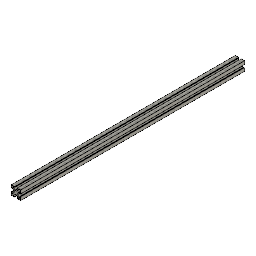
Frame Assembly v7 (Autodesk Fusion 360 archive; units mm, degrees)
design "TS10-10"
Autodesk Fusion 360 part; units mm, degrees
sketch "Sketch1" plane through (0, 0, 0) normal (0, 1, 0) x (1, 0, 0)
  line L0 (0, 0) -> (0, 4.826)
  line L1 (0, 4.826) -> (2, 4.826)
  line L2 (2, 4.826) -> (7.874, 10.7)
  line L3 (7.874, 10.7) -> (3.302, 10.7)
  line L4 (3.302, 10.7) -> (3.302, 12.7)
  line L5 (3.302, 12.7) -> (12.7, 12.7)
  line L6 (12.7, 12.7) -> (12.7, 3.302)
  line L7 (12.7, 3.302) -> (10.7, 3.302)
  line L8 (10.7, 3.302) -> (10.7, 7.874)
  line L9 (10.7, 7.874) -> (4.826, 2)
  line L10 (4.826, 2) -> (4.826, 0)
  line L11 (4.826, 0) -> (0, 0)
  line L12 (0, 4.826) -> (-2, 4.826)
  line L13 (-4.826, 2) -> (-4.826, 0)
  line L14 (-7.874, 10.7) -> (-3.302, 10.7)
  line L15 (-10.7, 3.302) -> (-10.7, 7.874)
  line L16 (-4.826, 0) -> (0, 0)
  line L17 (-12.7, 3.302) -> (-10.7, 3.302)
  line L18 (-3.302, 10.7) -> (-3.302, 12.7)
  line L19 (-2, 4.826) -> (-7.874, 10.7)
  line L20 (-12.7, 12.7) -> (-12.7, 3.302)
  line L21 (-3.302, 12.7) -> (-12.7, 12.7)
  line L22 (-10.7, 7.874) -> (-4.826, 2)
  line L23 (0, -4.826) -> (2, -4.826)
  line L24 (12.7, -3.302) -> (10.7, -3.302)
  line L25 (7.874, -10.7) -> (3.302, -10.7)
  line L26 (3.302, -10.7) -> (3.302, -12.7)
  line L27 (3.302, -12.7) -> (12.7, -12.7)
  line L28 (-12.7, -3.302) -> (-10.7, -3.302)
  line L29 (10.7, -7.874) -> (4.826, -2)
  line L30 (-10.7, -7.874) -> (-4.826, -2)
  line L31 (-10.7, -3.302) -> (-10.7, -7.874)
  line L32 (-12.7, -12.7) -> (-12.7, -3.302)
  line L33 (12.7, -12.7) -> (12.7, -3.302)
  line L34 (4.826, -2) -> (4.826, 0)
  line L35 (2, -4.826) -> (7.874, -10.7)
  line L36 (10.7, -3.302) -> (10.7, -7.874)
  line L37 (0, -4.826) -> (-2, -4.826)
  line L38 (-7.874, -10.7) -> (-3.302, -10.7)
  line L39 (-4.826, -2) -> (-4.826, 0)
  line L40 (-3.302, -10.7) -> (-3.302, -12.7)
  line L41 (0, 0) -> (0, -4.826)
  line L42 (-2, -4.826) -> (-7.874, -10.7)
  line L43 (-3.302, -12.7) -> (-12.7, -12.7)
  dimension "d1" = 12.7
  dimension "d2" = 12.7
  dimension "d3" = 3.302
  dimension "d4" = 3.302
  dimension "d5" = 7.874
  dimension "d6" = 7.874
  dimension "d8" = 7.874
  dimension "d9" = 2
  dimension "d10" = 2
  constraint coincident L0.start L11.end
  constraint vertical L0
  constraint perpendicular L0 L1
  constraint perpendicular L3 L4
  constraint perpendicular L4 L5
  constraint perpendicular L5 L6
  constraint perpendicular L4 L7
  constraint perpendicular L0 L11
  constraint vertical L10
  constraint coincident L3.end L4.start
  constraint coincident L7.end L8.start
  constraint vertical L8
  constraint equal L3 L8
  constraint parallel L2 L9
  constraint equal L1 L10
  constraint symmetric L11.end L0 L16.end
  constraint symmetric L1.start L0 L12.start
  constraint symmetric L0 L1.end L12.end
  constraint symmetric L0 L2.end L14.start
  constraint symmetric L0 L3.end L14.end
  constraint symmetric L0 L4.end L18.end
  constraint symmetric L0 L5.end L20.start
  constraint symmetric L0 L6.end L17.start
  constraint symmetric L0 L7.end L15.start
  constraint symmetric L0 L8.end L15.end
  constraint symmetric L0 L9.end L13.start
  constraint symmetric L0 L10.end L13.end
  constraint symmetric L0.start L11 L16.end
  constraint symmetric L0.end L11 L23.start
  constraint symmetric L1.end L11 L23.end
  constraint symmetric L2.end L11 L25.start
  constraint symmetric L3.end L11 L25.end
  constraint symmetric L4.end L11 L26.end
  constraint symmetric L5.end L11 L27.end
  constraint symmetric L6.end L11 L24.start
  constraint symmetric L7.end L11 L24.end
  constraint symmetric L8.end L11 L29.start
  constraint symmetric L9.end L11 L29.end
  constraint symmetric L10.end L11 L34.end
  constraint symmetric L11 L0.start L16.end
  constraint symmetric L11 L0.end L23.start
  constraint symmetric L11 L12.end L37.end
  constraint symmetric L11 L15.start L28.end
  constraint symmetric L11 L15.end L30.start
  constraint symmetric L11 L17.start L28.start
  constraint symmetric L11 L20.start L32.start
  constraint symmetric L11 L13.end L16.start
  constraint symmetric L11 L13.start L30.end
  constraint symmetric L11 L18.end L40.end
  constraint symmetric L11 L14.start L38.start
  constraint symmetric L11 L14.end L38.end
  measures "d1" horizontal distance of L0.start L5.end
  measures "d2" vertical distance of L0.start L5.end
  measures "d3" horizontal distance of L0.start L4.end
  measures "d4" vertical distance of L0.start L6.end
  measures "d5" distance of L1 L5
  measures "d6" distance of L6 L10
  measures "d8" horizontal distance of L0.start L2.end
  measures "d9" distance of L3.end L4.end
  measures "d10" distance of L6.end L7.end
extrude "Extrude1" add sketch "Sketch1" along normal blind 609.33
equation "d2 = d1"
equation "d3 = 0.26 in / 2"
equation "d4 = d3"
equation "d8 = 0.62 in / 2"

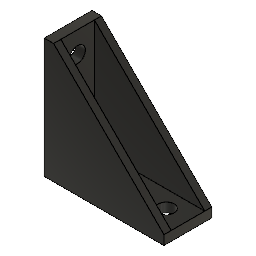
design "Small Bracket"
Autodesk Fusion 360 part; units mm, degrees
sketch "Sketch1" plane through (0, 0, 0) normal (0, 1, 0) x (1, 0, 0)
  line L0 (0, 0) -> (50, 0)
  line L1 (50, 0) -> (50, -4)
  line L2 (50, -4) -> (4, -4)
  line L3 (4, -4) -> (4, -50)
  line L4 (4, -50) -> (0, -50)
  line L5 (0, -50) -> (0, 0)
  line L6 (4, -50) -> (50, -4)
  dimension "d1" = 4
  dimension "d2" = 4
  dimension "d3" = 50
  dimension "d4" = 50
  constraint coincident L0.start L5.end
  constraint horizontal L0
  constraint perpendicular L0 L1
  constraint perpendicular L1 L2
  constraint perpendicular L2 L3
  constraint perpendicular L3 L4
  constraint perpendicular L0 L5
  measures "d1" distance of L0.end L1.end
  measures "d2" distance of L3.end L4.end
  measures "d3" distance of L4.end L0.start
  measures "d4" distance of L0.start L0.end
extrude "Extrude1" add sketch "Sketch1" along normal blind 20
extrude "Extrude2" cut sketch "Sketch1" along normal blind 17 contours L2 L3 L6
extrude "Extrude3" add sketch "Sketch1" along normal blind 3 contours L2 L3 L6
sketch "Sketch2" plane through (0, 0, 0) normal (0, 0, -1) x (1, 0, 0)
  line L0 (50, 0) -> (0, 0)
  line L1 (0, 0) -> (0, -20)
  line L2 (0, -20) -> (50, -20)
  line L3 (50, -20) -> (50, 0)
  point P0 (15, -10)
  point P1 (41, -10)
  dimension "d12" = 20
  dimension "d13" = 10
  dimension "d14" = 10
  dimension "d24" = 26
  dimension "d25" = 15
  measures "d12" distance of L0.end L1.end
  measures "d13" vertical distance of L0.end P0
  measures "d14" vertical distance of L0.end P1
  measures "d24" distance of P0 P1
  measures "d25" horizontal distance of L0.end P0
hole "Hole1" at (15, 10, 0) at (41, 10, 0) direction (0, 0, 1) diameter 6.5 depth 11 tip angle 180
sketch "Sketch3" plane through (0, 0, 0) normal (-1, 0, 0) x (0, -1, 0)
  line L0 (0, 0) -> (0, 50)
  line L1 (0, 50) -> (-20, 50)
  line L2 (-20, 50) -> (-20, 0)
  line L3 (-20, 0) -> (0, 0)
  point P0 (-10, 15)
  point P1 (-10, 41)
  dimension "d19" = 15
  dimension "d26" = 26
  measures "d19" vertical distance of L0.start P0
  measures "d26" distance of P0 P1
hole "Hole2" at (0, 10, 15) at (0, 10, 41) direction (1, 0, 0) diameter 6.5 depth 11 tip angle 180
equation "d13 = d12 / 2"
equation "d14 = d12 / 2"

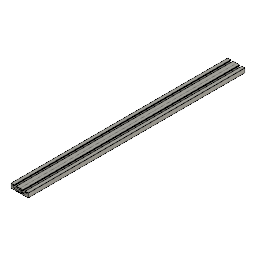
design "TS20-50-635"
Autodesk Fusion 360 part; units mm, degrees
sketch "Sketch1" plane through (0, 0, 0) normal (0, 1, 0) x (1, 0, 0)
  line L0 (0, 0) -> (25.4, 0)
  line L1 (-6.6089, -2) -> (0, -10.7)
  line L2 (9.398, -10.2) -> (9.398, -12.7)
  line L3 (-20.1422, -10.2) -> (-16.002, -4.7498)
  line L4 (25.4, -12.7) -> (16.002, -12.7)
  line L5 (-9.398, -10.2) -> (-9.398, -12.7)
  line L6 (-16.002, -12.7) -> (-16.002, -10.2)
  line L7 (0, 0) -> (0, -2)
  line L8 (9.398, -4.7498) -> (5.2578, -10.2)
  line L9 (16.002, -12.7) -> (16.002, -10.2)
  line L10 (0, 0) -> (-25.4, 0)
  line L11 (-5.2578, -10.2) -> (-9.398, -10.2)
  line L12 (-25.4, -12.7) -> (-16.002, -12.7)
  line L13 (-25.4, 0) -> (-25.4, -12.7)
  line L14 (0, -2) -> (6.6089, -2)
  line L15 (6.6089, -2) -> (0, -10.7)
  line L16 (-16.002, -10.2) -> (-20.1422, -10.2)
  line L17 (-9.398, -12.7) -> (0, -12.7)
  line L18 (0, -2) -> (-6.6089, -2)
  line L19 (-16.002, -4.7498) -> (-9.398, -4.7498)
  line L20 (16.002, -10.2) -> (20.1422, -10.2)
  line L21 (25.4, 0) -> (25.4, -12.7)
  line L22 (9.398, -12.7) -> (0, -12.7)
  line L23 (5.2578, -10.2) -> (9.398, -10.2)
  line L24 (20.1422, -10.2) -> (16.002, -4.7498)
  line L25 (16.002, -4.7498) -> (9.398, -4.7498)
  line L26 (-9.398, -4.7498) -> (-5.2578, -10.2)
  line L27 (0, -10.7) -> (0, -12.7)
  dimension "d1" = 12.7
  dimension "d2" = 2.5
  dimension "d3" = 6.604
  dimension "d4" = 6.604
  dimension "d5" = 14.8844
  dimension "d6" = 7.9502
  dimension "d7" = 25.4
  dimension "d8" = 9.398
  dimension "d9" = 2
  dimension "d10" = 2
  constraint horizontal L10
  constraint perpendicular L10 L13
  constraint perpendicular L12 L13
  constraint perpendicular L6 L12
  constraint perpendicular L6 L16
  constraint perpendicular L6 L19
  constraint parallel L11 L19
  constraint perpendicular L5 L11
  constraint perpendicular L5 L17
  constraint collinear L12 L17
  constraint collinear L11 L16
  constraint equal L11 L16
  constraint collinear L19.end L5.end L5.start
  constraint coincident L0.start L7.start
  constraint perpendicular L7 L17
  constraint perpendicular L7 L18
  constraint coincident L1.end L7
  constraint parallel L1 L26
  constraint collinear L7 L27
  constraint symmetric L0.start L10.start L7
  constraint symmetric L0.end L10.end L7
  constraint symmetric L4.start L12.start L7
  constraint symmetric L4.end L6.start L7
  constraint symmetric L9.end L6.end L7
  constraint symmetric L20.end L3.start L7
  constraint symmetric L24.end L3.end L7
  constraint symmetric L8.start L19.end L7
  constraint symmetric L8.end L11.start L7
  constraint symmetric L2.start L5.start L7
  constraint symmetric L2.end L5.end L7
  constraint symmetric L17.end L22.end L7
  constraint symmetric L14.start L18.start L7
  constraint symmetric L1.start L14.end L7
  constraint symmetric L1.end L15.end L7
  measures "d1" distance of L10 L12
  measures "d2" distance of L12 L16
  measures "d3" distance of L6.start L5.end
  measures "d4" distance of L3.end L19.end
  measures "d5" distance of L3.start L11.start
  measures "d6" vertical distance of L3.end L6.start
  measures "d7" distance of L0.start L13
  measures "d8" horizontal distance of L0.start L5.end
  measures "d9" distance of L7.end L0.start
  measures "d10" distance of L17.end L1.end
extrude "Extrude1" add sketch "Sketch1" along normal blind 635.4 contours L0 L2 L4 L7 L8 L9 L14 L15 L20 L21 L22 L23 L24 L25 L27 | L1 L3 L5 L6 L7 L10 L11 L12 L13 L16 L17 L18 L19 L26 L27
equation "d8 = d7 / 2 - d3 / 2"
equation "d11 = 610 mm + 12.7 mm * 2"

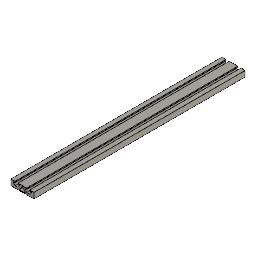
design "TS20-50-459"
Autodesk Fusion 360 part; units mm, degrees
sketch "Sketch1" plane through (0, 0, 0) normal (0, 1, 0) x (1, 0, 0)
  line L0 (0, 0) -> (-25.4, 0)
  line L1 (-25.4, 0) -> (-25.4, -12.7)
  line L2 (-25.4, -12.7) -> (-16.002, -12.7)
  line L3 (-16.002, -12.7) -> (-16.002, -10.2)
  line L4 (-16.002, -10.2) -> (-20.1422, -10.2)
  line L5 (-20.1422, -10.2) -> (-16.002, -4.7498)
  line L6 (-16.002, -4.7498) -> (-9.398, -4.7498)
  line L7 (-9.398, -4.7498) -> (-5.2578, -10.2)
  line L8 (-5.2578, -10.2) -> (-9.398, -10.2)
  line L9 (-9.398, -10.2) -> (-9.398, -12.7)
  line L10 (-9.398, -12.7) -> (0, -12.7)
  line L11 (0, -2) -> (-6.6089, -2)
  line L12 (-6.6089, -2) -> (0, -10.7)
  line L13 (0, 0) -> (0, -2)
  line L14 (0, -10.7) -> (0, -12.7)
  line L15 (9.398, -10.2) -> (9.398, -12.7)
  line L16 (16.002, -4.7498) -> (9.398, -4.7498)
  line L17 (16.002, -12.7) -> (16.002, -10.2)
  line L18 (5.2578, -10.2) -> (9.398, -10.2)
  line L19 (20.1422, -10.2) -> (16.002, -4.7498)
  line L20 (25.4, 0) -> (25.4, -12.7)
  line L21 (9.398, -12.7) -> (0, -12.7)
  line L22 (16.002, -10.2) -> (20.1422, -10.2)
  line L23 (0, 0) -> (25.4, 0)
  line L24 (6.6089, -2) -> (0, -10.7)
  line L25 (9.398, -4.7498) -> (5.2578, -10.2)
  line L26 (0, -2) -> (6.6089, -2)
  line L27 (25.4, -12.7) -> (16.002, -12.7)
  dimension "d1" = 12.7
  dimension "d2" = 2.5
  dimension "d3" = 6.604
  dimension "d4" = 6.604
  dimension "d5" = 14.8844
  dimension "d6" = 7.9502
  dimension "d7" = 25.4
  dimension "d8" = 9.398
  dimension "d9" = 2
  dimension "d10" = 2
  constraint horizontal L0
  constraint perpendicular L0 L1
  constraint perpendicular L1 L2
  constraint perpendicular L2 L3
  constraint perpendicular L3 L4
  constraint perpendicular L3 L6
  constraint parallel L6 L8
  constraint perpendicular L8 L9
  constraint perpendicular L9 L10
  constraint collinear L2 L10
  constraint collinear L4 L8
  constraint equal L4 L8
  constraint collinear L6.end L8.end L9.end
  constraint coincident L0.start L13.start
  constraint perpendicular L10 L13
  constraint perpendicular L11 L13
  constraint coincident L12.end L13
  constraint parallel L7 L12
  constraint collinear L13 L14
  constraint symmetric L0.start L13 L23.start
  constraint symmetric L0.end L13 L20.start
  constraint symmetric L1.end L13 L20.end
  constraint symmetric L2.end L13 L17.start
  constraint symmetric L3.end L13 L17.end
  constraint symmetric L4.end L13 L19.start
  constraint symmetric L5.end L13 L16.start
  constraint symmetric L6.end L13 L16.end
  constraint symmetric L7.end L13 L18.start
  constraint symmetric L8.end L13 L15.start
  constraint symmetric L9.end L13 L15.end
  constraint symmetric L10.end L13 L14.end
  constraint symmetric L11.start L13 L26.start
  constraint symmetric L11.end L13 L24.start
  constraint symmetric L12.end L13 L14.start
  measures "d1" distance of L0 L2
  measures "d2" distance of L2 L4
  measures "d3" distance of L2.end L9.end
  measures "d4" distance of L5.end L6.end
  measures "d5" distance of L4.end L7.end
  measures "d6" vertical distance of L2.end L5.end
  measures "d7" distance of L0.start L1
  measures "d8" horizontal distance of L0.start L9.end
  measures "d9" distance of L0.start L11.start
  measures "d10" distance of L10.end L12.end
extrude "Extrude1" add sketch "Sketch1" along normal blind 459 contours L0 L1 L2 L3 L4 L5 L6 L7 L8 L9 L10 L11 L12 L13 L14 | L13 L14 L15 L16 L17 L18 L19 L20 L21 L22 L23 L24 L25 L26 L27
equation "d8 = d7 / 2 - d3 / 2"
